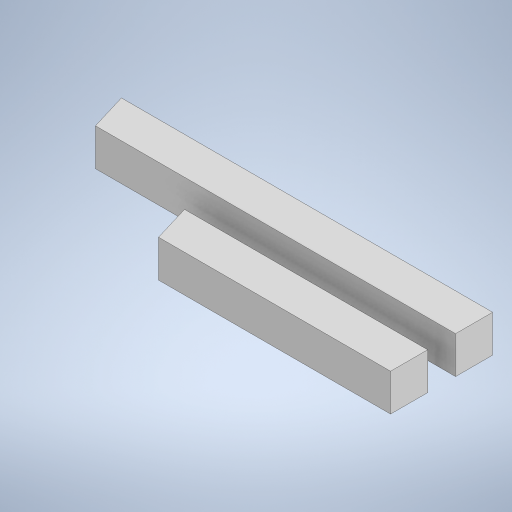
# Autodesk Inventor part: Bedienfeld_Fuesse
Saved by Autodesk Inventor 2023.1 (Build 271208000, 208)
## iProperties
Created: 2023-04-27
Part Number: Bedienfeld_Fuesse
Material: Generisch
Document SubType Name: Sheet Metal
Designer: marco
Density: 1 g/cm^3
Sheet Metal Rule: Standard_mm
Appearance: Vorgabe
Author: marco
Autodesk Inventor part; units mm, degrees
ref_plane "YZ Plane" through (0, 0, 0) normal (1, 0, 0) x (0, 1, 0)
ref_plane "XZ Plane" through (0, 0, 0) normal (0, 1, 0) x (-1, 0, 0)
ref_plane "XY Plane" through (0, 0, 0) normal (0, 0, 1) x (1, 0, 0)
sketch "Skizze1" plane through (0, 0, 0) normal (0, 1, 0) x (-1, 0, 0)
  line L0 (0, 0) -> (25, 0)
  line L1 (0, 0) -> (0, -50)
  line L2 (0, -50) -> (40, -50)
  line L3 (40, -50) -> (25, 0)
  line L4 (0, 0) -> (0, -4)
  line L5 (0, -4) -> (26.2, -4)
  line L6 (0, -50) -> (0, -46)
  line L7 (0, -46) -> (38.8, -46)
  line L8 (26.2, -4) -> (26.2, -46)
  line L9 (0, -46) -> (0, -43)
  line L10 (0, -43) -> (26.2, -43)
  line L11 (0, -43) -> (0, -39)
  line L12 (0, -39) -> (25, -39)
  line L13 (25, -39) -> (26.2, -43)
  dimension "d0" = 25
  dimension "d1" = 50
  dimension "d2" = 40
  dimension "d3" = 90
  dimension "d4" = 4
  dimension "d5" = 4
  dimension "d6" = 3
  dimension "d7" = 4
  dimension "d8" = 25
  dimension "d9" = 106.699
  dimension "d10" = 106.699
  constraints: 28 end point, 8 point on line, 6 perpendicular, 1 horizontal, 1 vertical
  measures "d0" distance of L0.start L0.end
  measures "d1" distance of L0.start L1.end
  measures "d2" distance of L1.end L2.end
  measures "d3" angle of L2 L1
  measures "d4" distance of L0.start L4.end
  measures "d5" distance of L1.end L6.end
  measures "d6" distance of L6.end L9.end
  measures "d7" distance of L9.end L11.end
  measures "d8" distance of L11.end L12.end
  measures "d9" angle of L12 L13
  measures "d10" angle of L0 L3
extrude "Extrusion1" add sketch "Skizze1" along normal blind 4 contours L12 L13 L10 L1 | L3 L2 L1 L7
equation "\"Biegeradius\" = Stärke"
equation "\"BreiteBiegungsfreistellung\" = Stärke"
equation "\"TiefeBiegungsfreistellung\" = 0.5 * Stärke"
equation "\"GrößeEckenfreistellung\" = 4 * Stärke"
equation "\"MinimalRest\" = 2 * Stärke"
equation "\"Übergangsradius\" = Biegeradius"
equation "\"JacobiRadiusGröße\" = Biegeradius"
equation "\"Abstandsgröße\" = Stärke"
equation "\"Stärke\" = 0.5"
